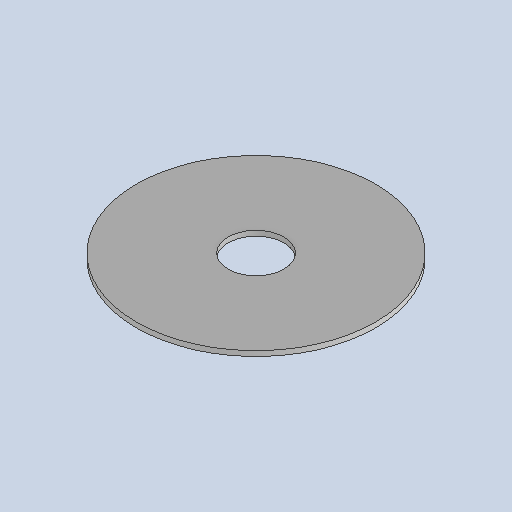
# Autodesk Inventor part: ДМС 040 лицо крышка
Saved by Autodesk Inventor 2024.2 (Build 282272000, 272)
## iProperties
Created: 2024-04-23
Part Number: ДМС 040 лицо крышка
Material: Generic
Document SubType Name: Modeling
Designer: admin
Density: 1 g/cm^3
Appearance: Default
Author: admin
Autodesk Inventor part; units mm, degrees
ref_plane "YZ Plane" through (0, 0, 0) normal (1, 0, 0) x (0, 1, 0)
ref_plane "XZ Plane" through (0, 0, 0) normal (0, 1, 0) x (-1, 0, 0)
ref_plane "XY Plane" through (0, 0, 0) normal (0, 0, 1) x (1, 0, 0)
sketch "Sketch1" plane through (0, 0, 0) normal (0, 0, 1) x (1, 0, 0)
  circle A0 centre (0, 0) radius 200 construction
  circle A1 centre (0, 0) radius 236
  circle A2 centre (0, 0) radius 55
  line L0 (0, 236) -> (0, 200)
  point P0 (0, 218)
  dimension "d0" = 400
  dimension "d4" = 110
  dimension "d12" = 36
  constraints: 3 coincident, 3 vertical alignment, 2 end point, 1 centre point, 1 midpoint, 1 vertical, 4 other
  measures "d4" diameter of A2
  measures "d12" distance of L0.start L0.end
extrude "Extrusion1" add sketch "Sketch1" along normal blind 10
equation "\"d0\" = Шпил_пласт_диам_центров"
equation "\"d4\" = Диам_отв_крышка_грязи"
equation "\"Шпил_пласт_диам_центров\" = 400"
equation "\"Диам_отв_крышка_грязи\" = 110"
body "Solid1"
